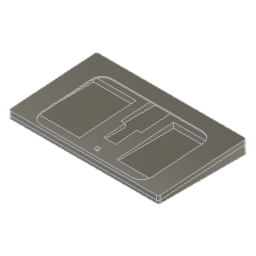
enclosure (Autodesk Fusion 360 design; units mm, degrees)
Autodesk Fusion 360 part; units mm, degrees
note: some values were not read from the file. Chosen so that the rebuilt part matches the saved one: a direction; which face or edge a step refers to; which pieces of a blend or face edit are solid. Set by a fixed rule: which sketch regions a step uses.
ref_plane "WorkPlane1" through (12.125, 0, 0) normal (0, -0.069756, 0.997564) x (1, 0, 0)
sketch "base" plane through (0, 0, 0) normal (0, -0.069756, 0.997564) x (1, 0, 0)
  line L0 (0, 82.5) -> (140, 82.5)
  line L1 (140, 82.5) -> (140, 0)
  line L2 (140, 0) -> (0, 0)
  line L3 (0, 0) -> (0, 82.5)
  dimension "d181" = 140
  dimension "d182" = 82.5
  constraint horizontal L0
  constraint vertical L1
  constraint horizontal L2
  constraint vertical L3
  constraint coincident L2.end L3.start
  measures "d181" distance of L0.start L0.end
  measures "d182" distance of L0.start L2.end
extrude "Extrude22" add sketch "base" against normal blind 2.5 makes body 1
sketch "surface" plane through (0, 0, 0) normal (0, -0.069756, 0.997564) x (-1, 0, 0)
  line L0 (-70, -82.5) -> (-70, 0) construction
  circle A0 centre (-44.9, -75.5) radius 1.5
  circle A1 centre (-44.9, -75.5) radius 1.75
  circle A2 centre (-5, -26) radius 1.5
  circle A3 centre (-5, -26) radius 1.75
  circle A4 centre (-5, -18) radius 1.5
  circle A5 centre (-5, -18) radius 1.75
  line L1 (-2.5, -30) -> (-2.5, -14)
  line L2 (0, -3.5) -> (-70, -3.5)
  line L3 (-37, -80) -> (-37, -72)
  line L4 (-37, -72) -> (-42, -72)
  line L5 (-42, -72) -> (-42, -80)
  line L6 (-65, -82.5) -> (-65, -80)
  line L7 (-60.5, -80) -> (-60.5, -44.5)
  line L8 (-64.5, -44.5) -> (-64.5, -24.5)
  line L9 (-64.5, -24.5) -> (-70, -24.5)
  circle A6 centre (-95.1, -75.5) radius 1.75
  circle A7 centre (-95.1, -75.5) radius 1.5
  circle A8 centre (-135, -26) radius 1.75
  circle A9 centre (-135, -26) radius 1.5
  circle A10 centre (-135, -18) radius 1.75
  circle A11 centre (-135, -18) radius 1.5
  line L10 (-75, -82.5) -> (-75, -80)
  line L11 (-79.5, -80) -> (-79.5, -44.5)
  line L12 (-79.5, -44.5) -> (-75.5, -44.5)
  line L13 (-75.5, -44.5) -> (-75.5, -24.5)
  line L14 (-75.5, -24.5) -> (-70, -24.5)
  line L15 (-98, -72) -> (-98, -80)
  line L16 (-103, -80) -> (-103, -72)
  line L17 (-103, -72) -> (-98, -72)
  line L18 (-137.5, -30) -> (-137.5, -14)
  line L19 (-140, -3.5) -> (-70, -3.5)
  line L20 (-68.5, -14.25) -> (-71.5, -14.25)
  line L21 (-71.5, -14.25) -> (-71.5, -11.25)
  line L22 (-71.5, -11.25) -> (-68.5, -11.25)
  line L23 (-68.5, -11.25) -> (-68.5, -14.25)
  line L24 (-12.5, -66.5) -> (-52.5, -66.5)
  line L25 (-52.5, -66.5) -> (-52.5, -13.5)
  line L26 (-52.5, -13.5) -> (-12.5, -13.5)
  line L27 (-12.5, -13.5) -> (-12.5, -66.5)
  line L28 (-127.5, -66.5) -> (-87.5, -66.5)
  line L29 (-87.5, -66.5) -> (-87.5, -13.5)
  line L30 (-127.5, -13.5) -> (-127.5, -66.5)
  line L31 (-87.5, -13.5) -> (-127.5, -13.5)
  line L32 (-5, -26) -> (-5, -18) construction
  line L33 (0, 0) -> (0, -82.5)
  line L34 (0, -82.5) -> (-140, -82.5)
  line L35 (-140, 0) -> (0, 0)
  line L36 (-140, -82.5) -> (-140, 0)
  line L37 (-60.5, -44.5) -> (-64.5, -44.5)
  circle A12 centre (-6, -76.5) radius 1.25
  circle A13 centre (-6, -76.5) radius 2
  circle A14 centre (-6, -8) radius 1.25
  circle A15 centre (-134, -76.5) radius 2
  circle A16 centre (-134, -76.5) radius 1.25
  circle A17 centre (-134, -8) radius 1.25
  circle A18 centre (-6, -8) radius 2
  circle A19 centre (-134, -8) radius 2
  line L38 (-2.5, -30) -> (-8.5, -30)
  line L39 (-8.5, -30) -> (-8.5, -14)
  line L40 (-8.5, -14) -> (-2.5, -14)
  line L41 (-2.5, -14) -> (-2.5, -30)
  line L42 (-137.5, -30) -> (-131.5, -30)
  line L43 (-131.5, -30) -> (-131.5, -14)
  line L44 (-131.5, -14) -> (-137.5, -14)
  line L45 (-70, -80) -> (-79.5, -80)
  line L46 (-98, -80) -> (-103, -80)
  line L47 (-70, -80) -> (-60.5, -80)
  line L48 (-42, -80) -> (-37, -80)
  dimension "d124" = 3
  dimension "d125" = 3.5
  dimension "d127" = 8
  dimension "d128" = 49.5
  dimension "d136" = 8
  dimension "d137" = 5
  dimension "d138" = 130
  dimension "d139" = 50.2
  dimension "d140" = 35.5
  dimension "d141" = 20
  dimension "d144" = 56
  dimension "d145" = 10
  dimension "d146" = 3
  dimension "d147" = 3
  dimension "d148" = 3.75
  dimension "d168" = 53
  dimension "d169" = 40
  dimension "d170" = 10
  dimension "d171" = 10
  dimension "d194" = 2.5
  dimension "d195" = 3.5
  dimension "d197" = 4.5
  dimension "d206" = 11
  dimension "d207" = 19
  dimension "d214" = 4
  dimension "d215" = 2.5
  dimension "d227" = 6
  dimension "d228" = 6
  dimension "d229" = 8
  dimension "d230" = 6
  dimension "d231" = 6
  dimension "d232" = 16
  dimension "d233" = 4
  dimension "d234" = 2.5
  constraint concentric A0 A1
  constraint concentric A2 A3
  constraint concentric A4 A5
  constraint equal A0 A2
  constraint equal A2 A4
  constraint equal A1 A3
  constraint equal A3 A5
  constraint coincident L0 L45.start
  constraint perpendicular L1 L47
  constraint coincident L0 L2.end
  constraint perpendicular L0 L2
  constraint perpendicular L3 L47
  constraint perpendicular L3 L4
  constraint coincident L5.end L47
  constraint perpendicular L5 L47
  constraint coincident L6.end L47
  constraint perpendicular L6 L47
  constraint perpendicular L7 L47
  constraint coincident L0 L9.end
  constraint perpendicular L0 L9
  constraint symmetric L0 A0 A7
  constraint symmetric L0 A1 A6
  constraint symmetric L0 A2 A9
  constraint symmetric L0 A3 A8
  constraint symmetric L0 A4 A11
  constraint symmetric L0 A5 A10
  constraint symmetric L0 L45.start L47.start
  constraint symmetric L0 L2.start L19.start
  constraint symmetric L0 L2.end L19.end
  constraint symmetric L0 L3.start L16.start
  constraint symmetric L0 L3.end L16.end
  constraint symmetric L0 L4.end L15.start
  constraint symmetric L0 L5.end L15.end
  constraint symmetric L0 L6.start L10.start
  constraint symmetric L0 L6.end L10.end
  constraint symmetric L0 L7.start L11.start
  constraint symmetric L0 L7.end L11.end
  constraint symmetric L0 L8.start L12.end
  constraint symmetric L0 L8.end L13.end
  constraint symmetric L0 L9.end L14.end
  constraint horizontal L20
  constraint vertical L21
  constraint horizontal L22
  constraint vertical L23
  constraint symmetric L0 L21 L23
  constraint horizontal L24
  constraint vertical L25
  constraint horizontal L26
  constraint vertical L27
  constraint symmetric L0 L24.start L28.start
  constraint symmetric L0 L24.end L28.end
  constraint symmetric L0 L25.end L29.end
  constraint symmetric L0 L26.end L30.start
  constraint coincident A2.centre A3.centre
  constraint coincident A4.centre A5.centre
  constraint vertical L32
  constraint perpendicular L0 L37
  constraint concentric A12 A13
  constraint symmetric L0 A12 A16
  constraint symmetric L0 A14 A17
  constraint midpoint L0.end L35
  constraint midpoint L0.start L34
  constraint coincident L6.start L34
  constraint concentric A14 A18
  constraint symmetric L0 A18 A19
  constraint equal A13 A18
  constraint equal A12 A14
  constraint symmetric L0 A13 A15
  constraint horizontal L38
  constraint vertical L39
  constraint horizontal L40
  constraint vertical L41
  constraint symmetric L0 L1.start L18.start
  constraint symmetric L0 L38.end L42.end
  constraint symmetric L0 L39.end L43.end
  constraint symmetric L0 L1.end L18.end
  constraint coincident L2.start L33
  constraint collinear L45 L46
  constraint collinear L47 L48
  measures "d124" diameter of A0
  measures "d125" diameter of A1
  measures "d127" distance of A2.centre A4.centre
  measures "d128" vertical distance of A0.centre A2.centre
  measures "d136" distance of L3.start L3.end
  measures "d137" distance of L3.end L4.end
  measures "d138" distance of A2.centre A8.centre
  measures "d139" distance of A0.centre A6.centre
  measures "d140" distance of L7.start L7.end
  measures "d141" distance of L8.start L8.end
  measures "d144" distance of L5 L15
  measures "d145" distance of L6 L10
  measures "d146" distance of L20.start L20.end
  measures "d147" distance of L20.start L22.end
  measures "d148" distance of A4.centre L20
  measures "d168" distance of L24.start L26.end
  measures "d169" distance of L24.start L24.end
  measures "d170" distance of L2 L26
  measures "d171" distance of L1 L27
  measures "d194" distance of L34 L47
  measures "d195" distance of L2 L35
  measures "d197" distance of A0.centre L47
  measures "d206" distance of L8 L13
  measures "d207" distance of L7 L11
  measures "d214" diameter of A13
  measures "d215" diameter of A12
  measures "d227" distance of L33 A12.centre
  measures "d228" distance of L34 A12.centre
  measures "d229" distance of L35 A14.centre
  measures "d230" distance of L33 A14.centre
  measures "d231" distance of L1.start L38.end
  measures "d232" distance of L1.start L1.end
  measures "d233" distance of A2.centre L38
  measures "d234" distance of L1 L33
ref_plane "WorkPlane2" through (70, 0.1744, -2.4939) normal (0, 0, 1) x (-1, 0, 0)
draft "Draft2" angle -4 neutral plane through (70, 0.1744, -2.4939) pull (0, 0, 1) 1 faces at (46.6667, 27.6074, -0.5756) on bodies 1
draft "Draft3" angle -4 neutral plane through (0, 0, 0) pull (0, 1, 0) 1 faces at (93.3333, 0.0581, -0.8313) on bodies 1
extrude "Extrude17" add sketch "surface" along normal blind 0.8 contours L20 L21 L22 L23 bodies 1
extrude "Extrude23" cut sketch "surface" along normal up to surface contours L7 L8 L9 L11 L12 L13 L14 L37 L45 L47 end surface through (0, 0.1744, -2.4939) normal (0, 0, -1) offset -2.5 bodies 1
extrude "Extrude15" cut sketch "surface" against normal blind 4 contours L6 L10 L34 L45 L47 bodies 1
extrude "Extrude18" cut sketch "surface" against normal blind 1.5 contours L3 L4 L5 L48 | L15 L16 L17 L46 bodies 1
extrude "Extrude19" cut sketch "surface" against normal through all contours A0 | A2 | A4 | A7 | A9 | A11 bodies 1
extrude "Extrude20" cut sketch "surface" against normal through all from surface at -2 contours A1 | A3 | A5 | A6 | A8 | A10 | A13 | A15 bodies 1
extrude "Extrude25" cut sketch "surface" against normal through all contours A12 | A13 | A14 | A15 | A16 | A17 | A18 | A19 bodies 1
extrude "Extrude29" add sketch "surface" against normal blind 1.5 contours A13 | A15 | A18 | A19 bodies 1
extrude "Extrude21" cut sketch "surface" along normal up to surface contours L24 L25 L26 L27 | L28 L29 L30 L31 end surface through (0, 0.1744, -2.4939) normal (0, 0, -1) offset -2 bodies 1
fillet "Fillet3" radius 2 4 edges at (140, 82.5874, 1.6305) (140, 0, -1.247) (0, 0, -1.247) (0, 82.5874, 1.6305) on bodies 1
fillet "Fillet4" radius 0.5 4 edges at (71.5, 14.1874, 1.3931) (71.5, 11.1947, 1.1838) (68.5, 11.1947, 1.1838) (68.5, 14.1874, 1.3931) on bodies 1
sketch "Sketch10" plane through (0, 0, 0) normal (0, -0.069756, 0.997564) x (1, 0, 0)
  line L0 (70, 82.5) -> (70, 0) construction
  line L1 (0, 82.5) -> (140, 82.5)
  line L2 (0, 0) -> (0, 82.5)
  line L3 (140, 0) -> (0, 0)
  line L4 (140, 82.5) -> (140, 0)
  line L5 (8.5, 30) -> (8.5, 14)
  line L6 (2.5, 30) -> (8.5, 30)
  line L7 (2.5, 30) -> (2.5, 14)
  line L8 (8.5, 14) -> (2.5, 14)
  circle A0 centre (6, 76.5) radius 0.75
  circle A1 centre (6, 8) radius 0.75
  line L9 (70, 80.7) -> (41, 80.7)
  line L10 (12.5, 79.5) -> (41, 79.5)
  line L11 (41, 79.5) -> (41, 80.7)
  line L12 (12.5, 79.5) -> (12.5, 30)
  line L13 (2.5, 30) -> (2.5, 14)
  line L14 (12.5, 14) -> (12.5, 3)
  line L15 (12.5, 13.5) -> (12.5, 66.5)
  line L16 (12.5, 30) -> (2.5, 30)
  line L17 (12.5, 14) -> (2.5, 14)
  line L18 (12.5, 3) -> (70, 3)
  line L19 (70, 80.7) -> (99, 80.7)
  line L20 (99, 79.5) -> (99, 80.7)
  line L21 (127.5, 79.5) -> (99, 79.5)
  line L22 (127.5, 79.5) -> (127.5, 30)
  line L23 (127.5, 30) -> (137.5, 30)
  line L24 (137.5, 30) -> (137.5, 14)
  line L25 (127.5, 14) -> (137.5, 14)
  line L26 (127.5, 14) -> (127.5, 3)
  line L27 (127.5, 3) -> (70, 3)
  circle A2 centre (134, 76.5) radius 0.75
  circle A3 centre (134, 76.5) radius 0.75
  circle A4 centre (134, 8) radius 0.75
  point P0 (6, 76.5)
  point P1 (6, 8)
  point P2 (134, 8)
  dimension "d241" = 1.5
  dimension "d242" = 1.5
  dimension "d243" = 29
  dimension "d244" = 1.8
  dimension "d245" = 3
  dimension "d246" = 3
  constraint coincident P0 A0.centre
  constraint coincident P1 A1.centre
  constraint coincident L0 L9.start
  constraint perpendicular L0 L9
  constraint perpendicular L2 L10
  constraint perpendicular L9 L11
  constraint coincident L6 L12.end
  constraint perpendicular L6 L12
  constraint coincident L6.start L7.start
  constraint coincident L7.end L8.end
  constraint coincident L8 L14.start
  constraint perpendicular L8 L14
  constraint collinear L12 L15
  constraint coincident L0 L18.end
  constraint perpendicular L0 L18
  constraint collinear L14 L15
  constraint symmetric L0 L9.start L19.start
  constraint symmetric L0 L9.end L19.end
  constraint symmetric L0 L10.start L21.start
  constraint symmetric L0 L10.end L20.start
  constraint symmetric L0 L12.end L22.end
  constraint symmetric L0 L6.start L23.end
  constraint symmetric L0 L7.end L24.end
  constraint symmetric L0 L14.start L25.start
  constraint symmetric L0 L14.end L26.end
  constraint symmetric L0 L18.end L27.end
  constraint symmetric L0 A0 A2
  constraint symmetric L0 P1 P2
  constraint symmetric L0 A0 A3
  constraint symmetric L0 A1 A4
  measures "d241" diameter of A0
  measures "d242" diameter of A1
  measures "d243" distance of L9.start L9.end
  measures "d244" distance of L1 L9
  measures "d245" distance of L1 L10
  measures "d246" distance of L3 L18
extrude "Extrude32" add sketch "Sketch10" along normal blind 3 separate body makes body 2
sketch "Sketch11" plane through (0, -0.2093, 2.9927) normal (0, -0.069756, 0.997564) x (1, 0, 0)
  circle A0 centre (6, 8) radius 0.75
  line L0 (137.5, 14) -> (127.5, 14)
  line L1 (127.5, 14) -> (127.5, 3)
  line L2 (127.5, 3) -> (12.5, 3)
  line L3 (12.5, 3) -> (12.5, 14)
  line L4 (12.5, 14) -> (2.5, 14)
  line L5 (2.5, 14) -> (2.5, 30)
  line L6 (2.5, 30) -> (12.5, 30)
  line L7 (12.5, 30) -> (12.5, 79.5)
  line L8 (12.5, 79.5) -> (41, 79.5)
  line L9 (41, 79.5) -> (41, 80.7)
  line L10 (41, 80.7) -> (99, 80.7)
  line L11 (99, 80.7) -> (99, 79.5)
  line L12 (99, 79.5) -> (127.5, 79.5)
  line L13 (127.5, 79.5) -> (127.5, 30)
  line L14 (127.5, 30) -> (137.5, 30)
  line L15 (137.5, 30) -> (137.5, 14)
  circle A1 centre (6, 76.5) radius 0.75
  circle A2 centre (134, 8) radius 0.75
  circle A3 centre (134, 76.5) radius 0.75
  line L16 (140, 82.5) -> (0, 82.5)
  line L17 (0, 82.5) -> (0, 0)
  line L18 (0, 0) -> (140, 0)
  line L19 (140, 0) -> (140, 82.5)
  line L20 (0, 82.5) -> (140, 82.5)
  line L21 (140, 82.5) -> (140, 0)
  line L22 (140, 0) -> (0, 0)
  line L23 (0, 0) -> (0, 82.5)
  line L24 (18, 59.5) -> (18, 12.5)
  line L25 (70, 82.5) -> (70, 0) construction
  line L26 (127.5, 3) -> (12.5, 3)
  arc A4 (18, 12.5) -> (27.5, 3) centre (27.5, 12.5) ccw
  line L27 (70, 3) -> (27.5, 3)
  line L28 (70, 69) -> (27.5, 69)
  arc A5 (27.5, 69) -> (18, 59.5) centre (27.5, 59.5) ccw
  line L29 (70, 69) -> (112.5, 69)
  arc A6 (122, 59.5) -> (112.5, 69) centre (112.5, 59.5) ccw
  line L30 (122, 59.5) -> (122, 12.5)
  arc A7 (112.5, 3) -> (122, 12.5) centre (112.5, 12.5) ccw
  line L31 (70, 3) -> (112.5, 3)
  dimension "d251" = 18
  dimension "d252" = 9.5
  dimension "d253" = 13.5
  constraint horizontal L20
  constraint vertical L21
  constraint horizontal L22
  constraint vertical L23
  constraint coincident L18.end L19.start
  constraint coincident L16.end L17.start
  constraint perpendicular L4 L24
  constraint midpoint L20 L25.start
  constraint midpoint L22 L25.end
  constraint coincident L2 A4.end
  constraint tangent L24 A4
  constraint midpoint L2 L27.start
  constraint tangent A4 L27
  constraint coincident L25 L28.start
  constraint perpendicular L25 L28
  constraint tangent L24 A5
  constraint tangent L28 A5
  constraint equal A4 A5
  constraint symmetric L24.start L25 A6.start
  constraint symmetric L24.end L25 L30.end
  constraint symmetric L25 A4.end A7.start
  constraint symmetric L25 A4 A7
  constraint symmetric L25 L27.start L31.start
  constraint symmetric L25 L28.start L29.start
  constraint symmetric L25 L28.end L29.end
  constraint symmetric L25 A5 A6
  measures "d251" distance of L23 L24
  measures "d252" radius of A4
  measures "d253" distance of L20 L28
extrude "Extrude33" add sketch "Sketch11" along normal blind 1 contours A0 | L0 L1 L2 L3 L4 L5 L6 L7 L8 L9 L10 L11 L12 L13 L14 L15 L24 L26 A4 L28 A5 L29 A6 L30 A7 | A1 | A2 | A3 | L16 L17 L18 L19 L20 L21 L22 L23 bodies 2
draft "Draft6" angle -4 neutral plane through (0, 0, 0) pull (0, 1, 0) 1 faces at (93.3333, -0.093, 1.3301) on bodies 2
fillet "Fillet5" radius 2 4 edges at (0, 82.1595, 7.75) (140, 82.1595, 7.75) (0, 0, 2.0049) (140, 0, 2.0049) on bodies 2
